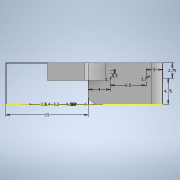
# Autodesk Inventor part: limit switch mount
Saved by Autodesk Inventor 2022 (Build 260153000, 153)
## iProperties
Created: 2022-02-19
Part Number: limit switch mount
Material: Generic
Document SubType Name: Modeling
Designer: a-dubs
Density: 1 g/cm^3
Appearance: Default
Author: a-dubs
Autodesk Inventor part; units mm, degrees
ref_plane "YZ Plane" through (0, 0, 0) normal (1, 0, 0) x (0, 1, 0)
ref_plane "XZ Plane" through (0, 0, 0) normal (0, 1, 0) x (-1, 0, 0)
ref_plane "XY Plane" through (0, 0, 0) normal (0, 0, 1) x (1, 0, 0)
sketch "Sketch1" plane through (0, 0, 0) normal (0, 0, 1) x (1, 0, 0)
  line L0 (0, 0) -> (6.5, 0)
  circle A0 centre (0, 0) radius 0.85
  circle A1 centre (6.5, 0) radius 0.85
  line L1 (0, 0) -> (-3, 0)
  line L2 (6.5, 0) -> (10.5, 0)
  line L3 (-3, 0) -> (-3, 4.75)
  line L4 (10.5, 0) -> (10.5, 4.75)
  line L5 (-3, 0) -> (-3, -2.75)
  line L6 (10.5, 0) -> (10.5, -2.75)
  line L7 (10.5, -2.75) -> (-3, -2.75)
  line L8 (-3, 4.75) -> (10.5, 4.75)
  line L9 (10.5, 4.75) -> (25.5, 4.75)
  line L10 (10.5, -2.75) -> (25.5, -2.75)
  line L11 (25.5, -2.75) -> (25.5, 4.75)
  line L12 (6.5, -0.85) -> (6.5, -1.35)
  line L13 (6.5, -1.35) -> (10.5, -1.35)
  line L14 (10.5, -1.35) -> (10.5, -2.75)
  line L15 (6.5, -1.35) -> (-3, -1.35)
  dimension "d2" = 1.7
  dimension "d0" = 6.5
  dimension "d1" = 1.7
  dimension "d3" = 3
  dimension "d4" = 4
  dimension "d5" = 4.75
  dimension "d6" = 2.75
  dimension "d9" = 15
  dimension "d10" = 0.5
  constraints: 32 end point, 6 horizontal, 4 perpendicular, 4 vertical, 2 coincident, 2 parallel, 2 point on line, 1 centre point, 1 collinear, 1 vertical alignment, 2 other
  measures "d0" distance of L0.start L0.end
  measures "d1" diameter of A0
  measures "d3" distance of L1.start L1.end
  measures "d4" distance of L2.start L2.end
  measures "d5" distance of L1.end L3.end
  measures "d6" distance of L1.end L5.end
  measures "d9" distance of L4.end L9.end
  measures "d10" distance of L12.start L12.end
extrude "Extrusion1" add sketch "Sketch1" along normal blind 4 contours L1 A0 L0 | L0 A0 L1 | A0 L1 L3 L8 L4 L2 A1 L0 | L0 A1 L12 L15 L5 L1 A0 | A1 L2 L0 | L0 L2 A1 | L2 L6 L13 L12 A1 | L15 L13 L6 L7 L5
extrude "Extrusion2" add sketch "Sketch1" along normal blind 2.9 from surface at 4 contours L15 L13 L6 L7 L5
extrude "Extrusion3" add sketch "Sketch1" along normal blind 0.5 from surface at 4 contours L1 A0 L0 | L0 A0 L1 | A1 L2 L0 | L0 L2 A1
fillet "Fillet1" radius 0.85 2 edges at (-0.85, 0, 4.5) (5.65, 0, 4.5)
mirror "Mirror1" about plane through (3.75, -2.05, 6.9) normal (0, 0, 1) of "Extrusion3", "Fillet1", "Extrusion2", "Extrusion1"
sketch "Sketch2" plane through (-3, -1.35, 4) normal (0, 1, 0) x (1, 0, 0)
  line L0 (0, 0) -> (0, -5.8) projected
  line L1 (0, 0) -> (0, -5.8)
  line L2 (13.5, -5.8) -> (0, -5.8) projected
  line L3 (0, -5.8) -> (13.5, -5.8)
  line L4 (13.5, 0) -> (13.5, -5.8) projected
  line L5 (13.5, -5.8) -> (13.5, 0)
  line L6 (13.5, 0) -> (0, 0)
  line L7 (0, -2.9) -> (13.5, -2.9)
  line L8 (0, -2.9) -> (1.8, -2.9)
  line L9 (13.5, -2.9) -> (1.7, -2.9)
  line L10 (13.5, -2.9) -> (11.7, -2.9)
  line L11 (0, -2.9) -> (11.8, -2.9)
  line L12 (6.25, -2.9) -> (5.7, -2.9)
  line L13 (6.25, -2.9) -> (6.8, -2.9)
  line L14 (0, -2.9) -> (0, -2.6)
  line L15 (0, -2.9) -> (0, -3.2)
  line L16 (0, -3.2) -> (13.5, -3.2)
  line L17 (13.5, -2.6) -> (0, -2.6)
  line L18 (0.7, -2.6) -> (0.7, -3.2)
  line L19 (1.8, -2.6) -> (1.8, -3.2)
  line L20 (5.7, -2.6) -> (5.7, -3.2)
  line L21 (6.8, -3.2) -> (6.8, -2.6)
  line L22 (10.7, -2.6) -> (10.7, -3.2)
  line L23 (11.8, -2.6) -> (11.8, -3.2)
  point P0 (3, 4)
  dimension "d16" = 1.8
  dimension "d17" = 11.8
  dimension "d18" = 1.8
  dimension "d19" = 11.8
  dimension "d20" = 0.55
  dimension "d21" = 0.55
  dimension "d22" = 0.3
  dimension "d23" = 0.3
  constraints: 42 end point, 23 point on line, 8 perpendicular, 4 equal length, 2 midpoint
  measures "d16" distance of L7.start L8.end
  measures "d17" distance of L7.end L9.end
  measures "d18" distance of L7.end L10.end
  measures "d19" distance of L7.start L11.end
  measures "d20" distance of L12.start L12.end
  measures "d21" distance of L12.start L13.end
  measures "d22" distance of L7.start L14.end
  measures "d23" distance of L7.start L15.end
extrude "Extrusion4" cut sketch "Sketch2" against normal through all contours L17 L19 L7 L18 | L7 L19 L16 L18 | L23 L7 L22 L17 | L17 L21 L7 L20 | L23 L16 L22 L7 | L7 L21 L16 L20
extrude "Extrusion5" add sketch "Sketch1" along normal up to surface (13.8 mm away) contours L4 L9 L11 L10 L6
extrude "Extrusion6" add sketch "Sketch1" along normal blind 6.4 from surface at 13.8 contours L4 L9 L11 L10 L6
extrude "Extrusion7" add sketch "Sketch1" against normal blind 6.4 contours L4 L9 L11 L10 L6
sketch "Sketch3" plane through (-3, 4.75, 4) normal (0, 1, 0) x (1, 0, 0)
  line L0 (13.5, 4) -> (0, 4) projected
  line L1 (0, -9.8) -> (13.5, -9.8) projected
  line L2 (13.5, 4) -> (13.5, -9.8)
  line L3 (13.5, 0) -> (13.5, -5.8) projected
  line L4 (13.5, -2.9) -> (28.5, -2.9)
  line L5 (28.5, -16.2) -> (28.5, 10.4) projected
  line L6 (13.5, -2.9) -> (14.5, -2.9)
  line L7 (14.5, -2.9) -> (17.7, -2.9)
  line L8 (17.7, -2.9) -> (17.7, 6.6835)
  circle A0 centre (17.7, 6.6835) radius 1.6
  line L9 (17.7, -2.9) -> (17.7, -12.4835)
  circle A1 centre (17.7, -12.4835) radius 1.6
  circle A2 centre (24.1, 6.6835) radius 1.6
  line L10 (24.1, -2.9) -> (24.1, 6.6835)
  line L11 (24.1, -2.9) -> (24.1, -12.4835)
  circle A3 centre (24.1, -12.4835) radius 1.6
  line L12 (17.7, -12.4835) -> (20.9, -12.4835)
  line L13 (20.9, -12.4835) -> (20.9, -16.2)
  line L14 (28.5, -16.2) -> (13.5, -16.2) projected
  line L15 (20.9, -12.4835) -> (20.9, 10.4)
  line L16 (13.5, 10.4) -> (28.5, 10.4) projected
  line L17 (13.5, -16.2) -> (13.5, 10.4)
  line L18 (20.9, 10.4) -> (13.5, 10.4)
  line L19 (17.7, -12.4835) -> (17.7, -15.6835)
  line L20 (17.7, -15.6835) -> (20.9, -15.6835)
  line L21 (17.7, -15.6835) -> (13.5, -15.6835)
  line L22 (13.5, -9.8) -> (13.5, -16.2) projected
  line L23 (17.7, 6.6835) -> (17.7, 9.8835)
  line L24 (17.7, 9.8835) -> (20.9, 9.8835)
  line L25 (17.7, 9.8835) -> (13.5, 9.8835)
  point P0 (3, 4)
  point P1 (12.5, -9.8)
  dimension "d32" = 1
  dimension "d33" = 3.2
  dimension "d34" = 9.5835
  dimension "d35" = 3.2
  dimension "d38" = 6.4
  dimension "d47" = 3.2
  dimension "d56" = 3.2
  dimension "d57" = 3.2
  constraints: 38 end point, 11 point on line, 4 centre point, 4 coincident, 4 vertical, 3 perpendicular, 2 collinear, 2 horizontal, 2 midpoint, 2 symmetric about line, 10 other
  measures "d32" distance of L4.start L6.end
  measures "d33" distance of L6.end L7.end
  measures "d34" distance of L7.end L8.end
  measures "d35" diameter of A0
  measures "d38" distance of L23.start A2.centre
  measures "d47" distance of L12.start L12.end
  measures "d56" distance of L12.start L19.end
  measures "d57" distance of L23.start L23.end
extrude "Extrusion8" cut sketch "Sketch3" against normal through all contours L23 L8 A0 | A0 L8 L23 | A1 L12 L9 | L9 L19 A1 | L12 A1 L19 | A2 | A3
fillet "Fillet2" radius 2 6 edges at (25.5, 1, 20.2) (10.5, 1, 20.2) (-3, 1, 13.8) (-3, 1, 0) (25.5, 1, -6.4) (10.5, 1, -6.4)
fillet "Fillet3" radius 0.4 4 edges at (13.1, 4.75, 16.4835) (13.1, 4.75, -2.6835) (19.5, 4.75, 16.4835) (19.5, 4.75, -2.6835)
extrude "Extrusion9" cut sketch "Sketch3" against normal through all contours L17 L16 L15 L24 L25 | L16 L5 L4 L15 | L4 L5 L14 L13 L15 | L21 L20 L13 L14 L17 | A2 | A3
extrude "Extrusion10" cut sketch "Sketch3" against normal blind 4.3 contours L17 L25 L23 A0 L8 L4 L2 | L17 L16 L15 L24 L25 | L4 L9 A1 L19 L21 L17 L2 | L24 L15 L4 L8 A0 L23 | L23 L8 A0 | A0 L8 L23 | L4 L15 L12 A1 L9 | L21 L20 L13 L14 L17 | A1 L12 L9 | L9 L19 A1 | L13 L20 L19 A1 L12 | L12 A1 L19
chamfer "Chamfer1" distance 1.1 angle 45 2 edges at (10.5, 4.75, 2) (10.5, 4.75, 11.8)
fillet "Fillet4" radius 2 2 edges at (9.4, 4.75, 2) (9.4, 4.75, 11.8)
fillet "Fillet5" radius 3.2 2 edges at (10.5, -1.15, 0) (10.5, -1.15, 13.8)
equation "\"d15\" = 0.5 * d1"
body "Solid1"
